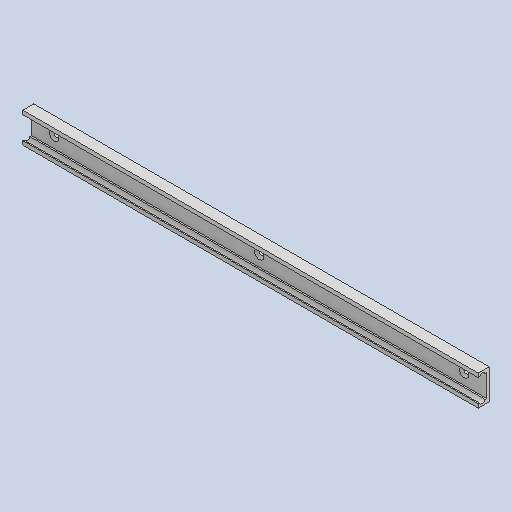
# Autodesk Inventor part: Outside
Saved by Autodesk Inventor 2022 (Build 260153000, 153)
## iProperties
Created: 2021-09-24
Part Number: Outside
Material: Generic
Document SubType Name: Modeling
Designer: deli
Density: 1 g/cm^3
Appearance: Default
Author: deli
Autodesk Inventor part; units mm, degrees
ref_plane "YZ Plane" through (0, 0, 0) normal (1, 0, 0) x (0, 1, 0)
ref_plane "XZ Plane" through (0, 0, 0) normal (0, 1, 0) x (-1, 0, 0)
ref_plane "XY Plane" through (0, 0, 0) normal (0, 0, 1) x (1, 0, 0)
sketch "Sketch1" plane through (0, 0, 0) normal (1, 0, 0) x (0, 1, 0)
  line L0 (50.6485, -6.1804) -> (53.2485, -6.1804)
  line L1 (53.2485, -6.1804) -> (53.2485, -13.3804)
  arc A0 (50.6485, -10.8603) -> (50.6485, -6.9005) centre (49.9485, -8.8804) ccw
  line L2 (50.6485, -6.1804) -> (50.6485, -6.9005)
  line L3 (50.6485, -10.8603) -> (50.6485, -11.8804)
  line L4 (50.6485, -11.8804) -> (35.8485, -11.8804)
  line L5 (53.2485, -13.3804) -> (33.2485, -13.3804)
  line L6 (33.2485, -13.3804) -> (33.2485, -6.1804)
  line L7 (33.2485, -6.1804) -> (35.8485, -6.1804)
  line L8 (35.8485, -6.1804) -> (35.8485, -6.9005)
  arc A1 (35.8485, -6.9005) -> (35.8485, -10.8603) centre (36.5485, -8.8804) ccw
  line L9 (35.8485, -10.8603) -> (35.8485, -11.8804)
  point P0 (0, 0)
  constraints: 20 end point, 4 point on circle, 2 centre point
extrude "Extrusion1" add sketch "Sketch1" along normal blind 300
sketch "Sketch2" plane through (0, 35.8485, -11.8804) normal (0, 0, 1) x (1, 0, 0)
  circle A0 centre (285, 7.4) radius 1.6 projected
  circle A1 centre (150, 7.4) radius 1.6 projected
  circle A2 centre (15, 7.4) radius 1.6 projected
  point P0 (0, -35.8485)
extrude "Extrusion2" cut sketch "Sketch2" against normal blind 300
chamfer "Chamfer1" distance 1.5 angle 45 3 edges at (13.4, 43.2485, -11.8804) (148.4, 43.2485, -11.8804) (283.4, 43.2485, -11.8804)
body "Solid1"
